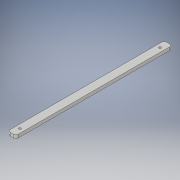
# Autodesk Inventor part: Lift
Saved by Autodesk Inventor 2019 (Build 230136000, 136)
## iProperties
Created: 2018-06-10
Part Number: Lift
Material: Ogólny
Document SubType Name: Modeling
Designer: Kamil
Density: 1 g/cm^3
Appearance: Domyślna
Author: Kamil
Autodesk Inventor part; units mm, degrees
ref_plane "YZ Plane" through (0, 0, 0) normal (1, 0, 0) x (0, 1, 0)
ref_plane "XZ Plane" through (0, 0, 0) normal (0, 1, 0) x (-1, 0, 0)
ref_plane "XY Plane" through (0, 0, 0) normal (0, 0, 1) x (1, 0, 0)
sketch "Szkic1" plane through (0, 0, 0) normal (0, 1, 0) x (-1, 0, 0)
  line L0 (2.5, 145) -> (-2.5, 145)
  line L1 (-7.5, 140) -> (-7.5, -140)
  line L2 (-2.5, -145) -> (2.5, -145)
  line L3 (7.5, -140) -> (7.5, 140)
  line L4 (7.5, 145) -> (-7.5, -145) construction
  line L5 (-7.5, 145) -> (7.5, -145) construction
  circle A0 centre (0, 130) radius 2
  circle A1 centre (0, -130) radius 2
  arc A2 (2.5, -145) -> (7.5, -140) centre (2.5, -140) ccw
  arc A3 (-7.5, -140) -> (-2.5, -145) centre (-2.5, -140) ccw
  arc A4 (7.5, 140) -> (2.5, 145) centre (2.5, 140) ccw
  arc A5 (-2.5, 145) -> (-7.5, 140) centre (-2.5, 140) ccw
  point P0 (0, 0)
  dimension "d0" = 15
  dimension "d1" = 290
  dimension "d2" = 4
  dimension "d3" = 4
  dimension "d4" = 5
  constraints: 12 end point, 8 point on circle, 8 point on line, 8 tangent, 6 centre point, 3 equal radius, 2 midpoint, 2 parallel, 1 horizontal, 1 perpendicular
  measures "d0" distance of L5.end L4.end
  measures "d1" distance of L4.end L5.start
  measures "d2" diameter of A0
  measures "d3" diameter of A1
  measures "d4" radius of A2
extrude "Wyciągnięcie proste1" add sketch "Szkic1" along normal blind 6
